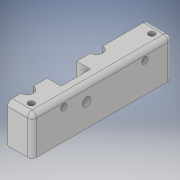
# Autodesk Inventor part: motorothersideradrod
Saved by Autodesk Inventor 2019.1 (Build 231200000, 200)
## iProperties
Created: 2019-08-05
Part Number: motorothersideradrod
Material: Generic
Document SubType Name: Modeling
Designer: rob
Density: 1 g/cm^3
Appearance: Default
Author: rob
## iProperties of the stored document motorothersideradrod_3DPrint.ipt
Created: 2019-08-13
Part Number: motorothersideradrod_3DPrint
Material: Generic
Document SubType Name: Modeling
Designer: Computus
Density: 1 g/cm^3
Appearance: Default
Author: Computus
Autodesk Inventor part; units mm, degrees
ref_plane "YZ Plane" through (0, 0, 0) normal (1, 0, 0) x (0, 1, 0)
ref_plane "XZ Plane" through (0, 0, 0) normal (0, 1, 0) x (-1, 0, 0)
ref_plane "XY Plane" through (0, 0, 0) normal (0, 0, 1) x (1, 0, 0)
sketch "Sketch1" plane through (0, 0, 0) normal (0, 1, 0) x (-1, 0, 0)
  line L0 (0, 0) -> (16, 0)
  line L1 (16, 0) -> (16, -91)
  line L2 (16, -91) -> (0, -91)
  line L3 (0, -91) -> (0, 0)
  dimension "d0" = 16
  dimension "d1" = 91
  constraints: 8 end point, 2 parallel, 1 horizontal, 1 perpendicular
  measures "d0" distance of L1.end L2.end
  measures "d1" distance of L0.end L1.end
extrude "Extrusion1" add sketch "Sketch1" along normal blind 25
sketch "Sketch2" plane through (0, 25, 0) normal (0, 1, 0) x (1, 0, 0)
  line L0 (-16, 91) -> (-16, 0) projected
  circle A0 centre (-16, 12.8045) radius 4
  circle A1 centre (-16, 57.8045) radius 4
  point P0 (0, 0)
  dimension "d4" = 8
  dimension "d5" = 8
  dimension "d6" = 45
  constraints: 2 centre point, 2 point on line
  measures "d4" diameter of A0
  measures "d5" diameter of A1
  measures "d6" distance of A1.centre A0.centre
extrude "Extrusion2" cut sketch "Sketch2" against normal blind 20
fillet "Fillet1" radius 3 5 edges at (0, 12.5, -91) (0, 12.5, 0) (0, 25, -45.5) (-8, 25, -91) (-8, 25, 0)
sketch "Sketch3" plane through (0, 25, 0) normal (0, 1, 0) x (1, 0, 0)
  circle A0 centre (-7, 6.5) radius 2
  circle A1 centre (-7, 84.5) radius 2
  line L0 (-16, 8.8045) -> (-16, 3) projected
  line L1 (-16, 53.8045) -> (-16, 16.8045) projected
  line L2 (-16, 88) -> (-16, 61.8045) projected
  point P0 (0, 0)
  dimension "d10" = 4
  dimension "d12" = 4
  dimension "d15" = 9
  dimension "d17" = 9
  dimension "d18" = 6.5
  constraints: 2 centre point
  measures "d10" diameter of A0
  measures "d12" diameter of A1
  measures "d15" distance from line of L0 A0.centre
  measures "d17" distance from line of L2 A1.centre
  measures "d18" vertical distance of point (0, 0) A0.centre
sketch "Sketch4" plane through (0, 0, -3) normal (1, 0, 0) x (0, 0, -1)
  circle A0 centre (17.4261, 19.4387) radius 2
  circle A1 centre (69.9995, 19.4387) radius 2
  point P0 (-3, 0)
  dimension "d21" = 4
  dimension "d22" = 4
  constraints: 2 centre point
  measures "d21" diameter of A0
  measures "d22" diameter of A1
extrude "Extrusion4" cut sketch "Sketch4" against normal blind 30
sketch "Sketch5" plane through (-16, 0, -91) normal (-1, 0, 0) x (0, 0, 1)
  point P0 (91, 0)
sketch "Sketch6" plane through (-16, 0, -91) normal (-1, 0, 0) x (0, 0, 1)
  arc A0 (46.1955, 15) -> (65.1955, 15) centre (55.6955, 15) ccw
  line L0 (37.1955, 25) -> (37.1955, 5) projected
  line L1 (37.1955, 25) -> (74.1955, 25) projected
  line L2 (46.1955, 15) -> (46.1955, 30.0529)
  line L3 (46.1955, 30.0529) -> (65.1955, 30.0529)
  line L4 (65.1955, 30.0529) -> (65.1955, 15)
  point P0 (91, 0)
  dimension "d25" = 19
  dimension "d26" = 18.5
  dimension "d27" = 10
  constraints: 6 end point, 2 point on circle, 1 centre point, 1 parallel
  measures "d25" diameter of A0
  measures "d26" distance from line of L0 A0.centre
  measures "d27" distance from line of L1 A0.centre
extrude "Extrusion5" cut sketch "Sketch6" against normal blind 9
sketch "Sketch7" plane through (-7, 0, -91) normal (-1, 0, 0) x (0, 0, 1)
  circle A0 centre (55.6955, 15) radius 2.75
  line L0 (37.1955, 25) -> (37.1955, 5) projected
  point P0 (91, 0)
  dimension "d30" = 5.5
  dimension "d31" = 18.5
  constraints: 1 centre point
  measures "d30" diameter of A0
  measures "d31" distance from line of L0 A0.centre
extrude "Extrusion6" cut sketch "Sketch7" against normal blind 30
extrude "Extrusion7" cut sketch "Sketch3" against normal blind 30
body "Solid1"
